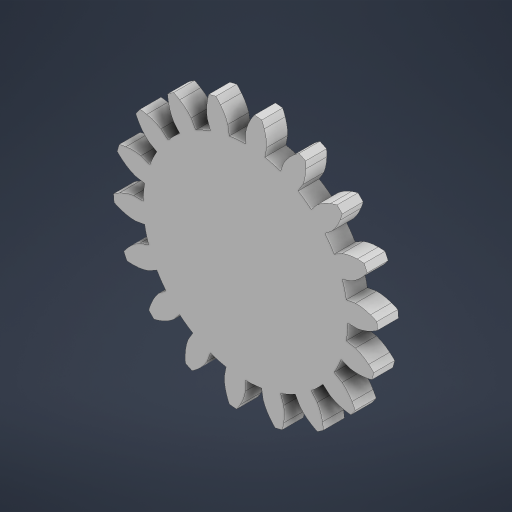
# Autodesk Inventor part: SpurGearTemplate
Saved by Autodesk Inventor 2024 (Build 280153000, 153)
## iProperties
Created: 2023-09-27
Part Number: SpurGearTemplate
Material: Generic
Document SubType Name: Modeling
Designer: avsar
Density: 1 g/cm^3
Appearance: Default
Author: avsar
Autodesk Inventor part; units mm, degrees
ref_plane "YZ Plane" through (0, 0, 0) normal (1, 0, 0) x (0, 1, 0)
ref_plane "XZ Plane" through (0, 0, 0) normal (0, 1, 0) x (-1, 0, 0)
ref_plane "XY Plane" through (0, 0, 0) normal (0, 0, 1) x (1, 0, 0)
sketch "Sketch1" plane through (0, 0, 0) normal (0, 0, 1) x (1, 0, 0)
  circle A0 centre (0, 0) radius 36 construction
  arc A1 (4.9129, 39.6971) -> (4.8245, 39.708) centre (0, 0) ccw
  arc A2 (31, 0) -> (5.8701, 30.4391) centre (0, 0) ccw construction
  circle A3 centre (0, 0) radius 32 construction
  circle A4 centre (0, 0) radius 33.8289 construction
  line L0 (0, 0) -> (0, 33.8289) construction
  line L1 (0, 0) -> (16.9145, 29.2967)
  line L2 (0, 0) -> (29.2967, 16.9145)
  line L3 (0, 0) -> (33.8289, 0)
  line L4 (33.8289, 0) -> (33.8289, 53.1384) construction
  line L5 (29.2967, 16.9145) -> (11.5839, 47.5939) construction
  line L6 (16.9145, 29.2967) -> (1.5747, 38.1531) construction
  arc A5 (1.5747, 38.1531) -> (0, 33.8289) centre (13.0619, 31.521) ccw
  arc A6 (11.5839, 47.5939) -> (3.9725, 41.5773) centre (22.3394, 26.1646) ccw construction
  arc A7 (33.8289, 53.1384) -> (11.5839, 47.5939) centre (35.0512, 0.8375) ccw construction
  line L7 (0, 0) -> (12.3127, 33.8289)
  line L8 (0, 0) -> (6.2513, 35.4531) construction
  arc A8 (6.2513, 35.4531) -> (0.5751, 35.9954) centre (0, 0) ccw construction
  line L9 (3.424, 35.8368) -> (0, 0) construction
  arc A9 (12.3127, 33.8289) -> (0.5751, 35.9954) centre (0, 0) ccw construction
  arc A10 (6.4058, 33.2169) -> (5.6784, 37.761) centre (-6.8568, 33.4241) ccw
  arc A11 (5.6784, 37.761) -> (4.9129, 39.6971) centre (-16.9807, 29.9214) ccw
  arc A12 (-2.362, 48.9264) -> (-23.1547, 58.5828) centre (-34.2584, 7.4597) ccw construction
  arc A13 (18.6243, 35.3997) -> (4.9129, 39.6971) centre (0, 0) ccw construction
  arc A14 (2.693, 39.9092) -> (18.6243, 35.3997) centre (0, 0) ccw construction
  arc A15 (3.9725, 41.5773) -> (2.693, 39.9092) centre (22.3394, 26.1646) ccw construction
  arc A16 (2.7819, 39.9031) -> (2.693, 39.9092) centre (0, 0) ccw
  arc A17 (4.8245, 39.708) -> (2.7819, 39.9031) centre (0, 0) ccw
  arc A18 (4.9129, 39.6971) -> (-2.362, 48.9264) centre (-16.9807, 29.9214) ccw construction
  arc A19 (2.693, 39.9092) -> (1.5747, 38.1531) centre (22.3394, 26.1646) ccw
  line L10 (6.4058, 33.2169) -> (0, 0) construction
  arc A20 (0, 31) -> (31, 0) centre (0, 0) ccw construction
  arc A21 (5.8701, 30.4391) -> (2.9484, 30.8595) centre (0, 0) ccw
  arc A22 (2.9484, 30.8595) -> (0, 31) centre (0, 0) ccw
  line L11 (0, 33.8289) -> (0, 31)
  line L12 (5.8701, 30.4391) -> (6.4058, 33.2169)
  dimension "BaseCircle" = 67.6579
  dimension "PitchCircle" = 72
  dimension "AddendumCircle" = 80
  dimension "RootCircle" = 62
  dimension "ClearanceCircle" = 64
  dimension "InvoluteControl" = 90
  dimension "BaseCircleQuarterCircumference" = 53.1384
  dimension "d10" = 35.4256
  dimension "d11" = 17.7128
  dimension "CircularPitch" = 20
  constraints: 50 point on circle, 26 end point, 22 centre point, 7 symmetric about line, 5 coincident, 5 point on line, 2 collinear, 2 concentric, 2 tangent, 2 vertical, 1 line through centre, 1 vertical alignment, 18 other
  measures "PitchCircle" diameter of A0
  measures "AddendumCircle" diameter of A1
  measures "RootCircle" diameter of A2
  measures "ClearanceCircle" diameter of A3
  measures "BaseCircleQuarterCircumference" distance of L3.end L4.end
  measures "d10" distance of L2.end L5.end
  measures "d11" distance of L1.end L6.end
  measures "CircularPitch" angle of L7 L0
extrude "Extrusion1" add sketch "Sketch1" along normal mid plane 6.35
pattern_circular "Circular Pattern1" count 18 over 360 about axis through (0, 0, -10) along (0, 0, 1) of "Extrusion1"
sketch "Sketch2" plane through (0, 0, 0) normal (0, 0, 1) x (1, 0, 0)
  arc A0 (0, 31) -> (31, 0) centre (0, 0) ccw construction
  circle A1 centre (0, 0) radius 31
  arc A2 (31, 0) -> (5.8701, 30.4391) centre (0, 0) ccw construction
  constraints: 1 centre point, 1 coincident, 1 concentric
extrude "Extrusion2" add sketch "Sketch2" along normal mid plane 6.35
equation "\"AddendumCircle\" = PitchCircle + 2 * Module"
equation "\"RootCircle\" = PitchCircle - 2.5 * Module"
equation "\"ClearanceCircle\" = PitchCircle - 2 * Module"
equation "\"BaseCircleQuarterCircumference\" = 0.785398 * BaseCircle"
equation "\"d10\" = 0.666667 * BaseCircleQuarterCircumference"
equation "\"d11\" = 0.333333 * BaseCircleQuarterCircumference"
equation "\"d18\" = GearThickness"
equation "\"PressureAngle\" = 20deg"
equation "\"Module\" = 4"
equation "\"GearThickness\" = 6.35"
body "Solid1"
